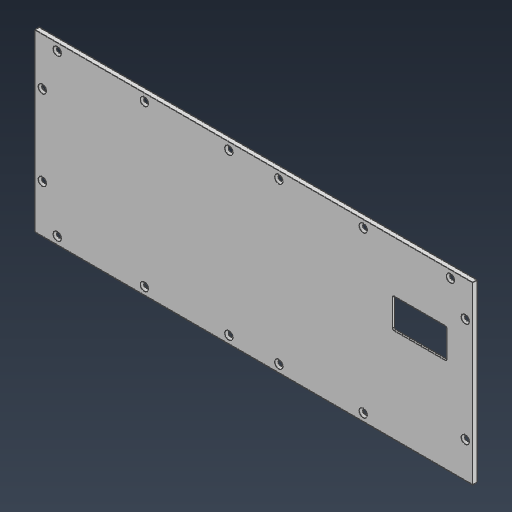
# Autodesk Inventor part: tpu_ceil
Saved by Autodesk Inventor 2023 (Build 270158000, 158)
## iProperties
Created: 2026-01-24
Part Number: tpu_ceil
Material: Generic
Document SubType Name: Modeling
Designer: szymo
Density: 1 g/cm^3
Appearance: Default
Author: szymo
Autodesk Inventor part; units mm, degrees
ref_plane "YZ Plane" through (0, 0, 0) normal (1, 0, 0) x (0, 1, 0)
ref_plane "Work Plane1" through (-125, 0, 3) normal (0, 0, 1) x (1, 0, 0)
sketch "Sketch1" plane through (-125, 0, 3) normal (0, 0, 1) x (1, 0, 0)
  circle A0 centre (241.5, 59.5) radius 1.5 projected
  circle A1 centre (163.8333, 91.5) radius 0.5 projected
  circle A2 centre (28.5, -91.5) radius 2.5 projected
  circle A3 centre (86.1667, -91.5) radius 0.5 projected
  circle A4 centre (125, 91.5) radius 1.5 projected
  circle A5 centre (241.5, 91.5) radius 0.5 projected
  circle A6 centre (241.5, 0) radius 0.5 projected
  circle A7 centre (241.5, -91.5) radius 0.5 projected
  circle A8 centre (28.5, 91.5) radius 1.5 projected
  circle A9 centre (125, -91.5) radius 1.5 projected
  circle A10 centre (86.1667, 91.5) radius 0.5 projected
  circle A11 centre (224.5, 91.5) radius 1.5 projected
  circle A12 centre (241.5, -59.5) radius 1.5 projected
  line L0 (151.825, -90.2) -> (140.325, -90.2) projected
  line L1 (151.825, -97.6) -> (151.825, -90.2) projected
  line L2 (140.325, -97.6) -> (151.825, -97.6) projected
  line L3 (140.325, -90.2) -> (140.325, -97.6) projected
  line L4 (250, -100) -> (0, -100) projected
  line L5 (250, 100) -> (250, -100) projected
  line L6 (0, 100) -> (250, 100) projected
  line L7 (0, 83) -> (0, 100) projected
  line L8 (233, 83) -> (0, 83) projected
  line L9 (233, -83) -> (233, 83) projected
  line L10 (0, -83) -> (233, -83) projected
  line L11 (0, -100) -> (0, -83) projected
  line L12 (197.325, -97.6) -> (208.825, -97.6) projected
  line L13 (197.325, -90.2) -> (197.325, -97.6) projected
  line L14 (208.825, -90.2) -> (197.325, -90.2) projected
  line L15 (208.825, -97.6) -> (208.825, -90.2) projected
  arc A13 (28.5, -96.5) -> (33.5, -91.5) centre (28.5, -91.5) ccw projected
  line L16 (33.5, -91.5) -> (33.5, 91.5) projected
  arc A14 (33.5, 91.5) -> (28.5, 96.5) centre (28.5, 91.5) ccw projected
  line L17 (28.5, 96.5) -> (-28.5, 96.5) projected
  arc A15 (-28.5, 96.5) -> (-33.5, 91.5) centre (-28.5, 91.5) ccw projected
  line L18 (-33.5, 91.5) -> (-33.5, -91.5) projected
  arc A16 (-33.5, -91.5) -> (-28.5, -96.5) centre (-28.5, -91.5) ccw projected
  line L19 (-28.5, -96.5) -> (28.5, -96.5) projected
  circle A17 centre (-28.5, 91.5) radius 1.5 projected
  circle A18 centre (-125, -91.5) radius 1.5 projected
  circle A19 centre (-241.5, 45.75) radius 1.5 projected
  circle A20 centre (-224.5, -91.5) radius 1.5 projected
  circle A21 centre (-241.5, -45.75) radius 1.5 projected
  circle A22 centre (-224.5, 91.5) radius 1.5 projected
  circle A23 centre (-28.5, -91.5) radius 1.5 projected
  circle A24 centre (-125, 91.5) radius 1.5 projected
  circle A25 centre (-163.8333, -91.5) radius 0.5 projected
  circle A26 centre (-241.5, 91.5) radius 0.5 projected
  circle A27 centre (-241.5, -91.5) radius 0.5 projected
  circle A28 centre (-86.1667, -91.5) radius 0.5 projected
  circle A29 centre (-241.5, 0) radius 0.5 projected
  circle A30 centre (-163.8333, 91.5) radius 0.5 projected
  circle A31 centre (-86.1667, 91.5) radius 0.5 projected
  line L20 (-250, 100) -> (-250, -100) projected
  line L21 (-250, -100) -> (0, -100) projected
  line L22 (0, -100) -> (0, -83) projected
  line L23 (0, -83) -> (-233, -83) projected
  line L24 (-233, -83) -> (-233, 83) projected
  line L25 (-233, 83) -> (0, 83) projected
  line L26 (0, 83) -> (0, 100) projected
  line L27 (0, 100) -> (-250, 100) projected
  arc A32 (-246.5, 45.75) -> (-239.7041, 41.0837) centre (-241.5, 45.75) ccw projected
  arc A33 (-239.7041, -41.0837) -> (-239.7041, 41.0837) centre (-233, 0) ccw projected
  arc A34 (-239.7041, -41.0837) -> (-246.5, -45.75) centre (-241.5, -45.75) ccw projected
  line L28 (-246.5, -45.75) -> (-246.5, -91.5) projected
  arc A35 (-246.5, -91.5) -> (-241.5, -96.5) centre (-241.5, -91.5) ccw projected
  line L29 (-241.5, -96.5) -> (-224.5, -96.5) projected
  arc A36 (-224.5, -96.5) -> (-219.5, -91.5) centre (-224.5, -91.5) ccw projected
  arc A37 (-157.8541, -15.573) -> (-219.5, -91.5) centre (-116.6841, -111.9884) ccw projected
  arc A38 (-130, -33.9663) -> (-157.8541, -15.573) centre (-150, -33.9663) ccw projected
  line L30 (-130, -33.9663) -> (-130, -91.5) projected
  arc A39 (-130, -91.5) -> (-120, -91.5) centre (-125, -91.5) ccw projected
  line L31 (-120, -91.5) -> (-120, 91.5) projected
  arc A40 (-120, 91.5) -> (-130, 91.5) centre (-125, 91.5) ccw projected
  line L32 (-130, 91.5) -> (-130, 33.9663) projected
  arc A41 (-157.8541, 15.573) -> (-130, 33.9663) centre (-150, 33.9663) ccw projected
  arc A42 (-219.5, 91.5) -> (-157.8541, 15.573) centre (-116.6841, 111.9884) ccw projected
  arc A43 (-219.5, 91.5) -> (-224.5, 96.5) centre (-224.5, 91.5) ccw projected
  line L33 (-224.5, 96.5) -> (-241.5, 96.5) projected
  arc A44 (-241.5, 96.5) -> (-246.5, 91.5) centre (-241.5, 91.5) ccw projected
  line L34 (-246.5, 91.5) -> (-246.5, 45.75) projected
  line L35 (-28.5, 97.5) -> (28.5, 97.5)
  arc A45 (34.5, 91.5) -> (28.5, 97.5) centre (28.5, 91.5) ccw
  line L36 (34.5, 91.5) -> (34.5, -91.5)
  arc A46 (28.5, -97.5) -> (34.5, -91.5) centre (28.5, -91.5) ccw
  line L37 (28.5, -97.5) -> (-28.5, -97.5)
  arc A47 (-34.5, -91.5) -> (-28.5, -97.5) centre (-28.5, -91.5) ccw
  line L38 (-34.5, -91.5) -> (-34.5, 91.5)
  arc A48 (-28.5, 97.5) -> (-34.5, 91.5) centre (-28.5, 91.5) ccw
  arc A49 (246.5, -59.5) -> (241.5, -54.5) centre (241.5, -59.5) ccw projected
  arc A50 (241.5, 54.5) -> (241.5, -54.5) centre (335.2622, 0) ccw projected
  arc A51 (241.5, 54.5) -> (246.5, 59.5) centre (241.5, 59.5) ccw projected
  line L39 (246.5, 59.5) -> (246.5, 91.5) projected
  arc A52 (246.5, 91.5) -> (241.5, 96.5) centre (241.5, 91.5) ccw projected
  line L40 (241.5, 96.5) -> (224.5, 96.5) projected
  arc A53 (224.5, 96.5) -> (219.5, 91.5) centre (224.5, 91.5) ccw projected
  arc A54 (130, 91.5) -> (219.5, 91.5) centre (174.75, 149.1692) ccw projected
  arc A55 (130, 91.5) -> (120, 91.5) centre (125, 91.5) ccw projected
  line L41 (120, 91.5) -> (120, -91.5) projected
  arc A56 (120, -91.5) -> (130, -91.5) centre (125, -91.5) ccw projected
  arc A57 (184.1388, -71.3462) -> (130, -91.5) centre (241.5, -308.2269) ccw projected
  arc A58 (236.5, -91.5) -> (184.1388, -71.3462) centre (176.2202, -170.0154) ccw projected
  arc A59 (236.5, -91.5) -> (246.5, -91.5) centre (241.5, -91.5) ccw projected
  line L42 (246.5, -91.5) -> (246.5, -59.5) projected
  line L43 (-119, 91.5) -> (-119, -91.5)
  arc A60 (-131, -91.5) -> (-119, -91.5) centre (-125, -91.5) ccw
  line L44 (-131, -91.5) -> (-131, -33.9663)
  arc A61 (-131, -33.9663) -> (-157.4614, -16.4927) centre (-150, -33.9663) ccw
  arc A62 (-157.4614, -16.4927) -> (-218.5009, -91.6034) centre (-116.6841, -111.9884) ccw
  arc A63 (-224.5, -97.5) -> (-218.5009, -91.6034) centre (-224.5, -91.5) ccw
  line L45 (-224.5, -97.5) -> (-241.5, -97.5)
  arc A64 (-247.5, -91.5) -> (-241.5, -97.5) centre (-241.5, -91.5) ccw
  line L46 (-247.5, -91.5) -> (-247.5, -45.75)
  arc A65 (-239.4465, -40.1124) -> (-247.5, -45.75) centre (-241.5, -45.75) ccw
  arc A66 (-239.4465, -40.1124) -> (-239.4465, 40.1124) centre (-233, 0) ccw
  arc A67 (-247.5, 45.75) -> (-239.4465, 40.1124) centre (-241.5, 45.75) ccw
  line L47 (-247.5, 45.75) -> (-247.5, 91.5)
  arc A68 (-241.5, 97.5) -> (-247.5, 91.5) centre (-241.5, 91.5) ccw
  line L48 (-241.5, 97.5) -> (-224.5, 97.5)
  arc A69 (-218.5009, 91.6034) -> (-224.5, 97.5) centre (-224.5, 91.5) ccw
  arc A70 (-218.5009, 91.6034) -> (-157.4614, 16.4927) centre (-116.6841, 111.9884) ccw
  arc A71 (-157.4614, 16.4927) -> (-131, 33.9663) centre (-150, 33.9663) ccw
  line L49 (-131, 33.9663) -> (-131, 91.5)
  arc A72 (-119, 91.5) -> (-131, 91.5) centre (-125, 91.5) ccw
  line L50 (119, -91.5) -> (119, 91.5)
  arc A73 (130.9784, 92.0084) -> (119, 91.5) centre (125, 91.5) ccw
  arc A74 (130.9784, 92.0084) -> (218.5216, 92.0084) centre (174.75, 149.1692) ccw
  arc A75 (224.5, 97.5) -> (218.5216, 92.0084) centre (224.5, 91.5) ccw
  line L51 (224.5, 97.5) -> (241.5, 97.5)
  arc A76 (247.5, 91.5) -> (241.5, 97.5) centre (241.5, 91.5) ccw
  line L52 (247.5, 91.5) -> (247.5, 59.5)
  arc A77 (242.0941, 53.5295) -> (247.5, 59.5) centre (241.5, 59.5) ccw
  arc A78 (242.0941, 53.5295) -> (242.0941, -53.5295) centre (335.2622, 0) ccw
  arc A79 (247.5, -59.5) -> (242.0941, -53.5295) centre (241.5, -59.5) ccw
  line L53 (247.5, -59.5) -> (247.5, -91.5)
  arc A80 (235.5218, -92.0111) -> (247.5, -91.5) centre (241.5, -91.5) ccw
  arc A81 (235.5218, -92.0111) -> (184.2182, -72.3559) centre (176.2202, -170.0154) ccw
  arc A82 (184.2182, -72.3559) -> (130.9671, -92.1278) centre (241.5, -308.2269) ccw
  arc A83 (119, -91.5) -> (130.9671, -92.1278) centre (125, -91.5) ccw
  circle A84 centre (-28.5, 91.5) radius 4 projected
  circle A85 centre (28.5, -91.5) radius 4 projected
  circle A86 centre (-28.5, -91.5) radius 4 projected
  circle A87 centre (28.5, 91.5) radius 4 projected
  circle A88 centre (-224.5, -91.5) radius 4 projected
  circle A89 centre (-241.5, 45.75) radius 4 projected
  circle A90 centre (-125, 91.5) radius 4 projected
  circle A91 centre (-224.5, 91.5) radius 4 projected
  circle A92 centre (-241.5, -45.75) radius 4 projected
  circle A93 centre (-125, -91.5) radius 4 projected
  circle A94 centre (224.5, 91.5) radius 4 projected
  circle A95 centre (125, -91.5) radius 4 projected
  circle A96 centre (241.5, -59.5) radius 4 projected
  circle A97 centre (125, 91.5) radius 4 projected
  circle A98 centre (241.5, 59.5) radius 4 projected
  circle A99 centre (176.2202, -33.9663) radius 26.1144 projected
  circle A100 centre (145.1053, 56.1526) radius 12.5237 projected
  arc A101 (161.2469, 11.514) -> (162.4469, 10.314) centre (162.4469, 11.514) ccw projected
  line L54 (161.2469, 11.514) -> (161.2469, 19.064) projected
  line L55 (161.2469, 19.064) -> (159.9469, 19.064) projected
  line L56 (159.9469, 19.064) -> (159.9469, 29.964) projected
  line L57 (159.9469, 29.964) -> (161.2469, 29.964) projected
  line L58 (161.2469, 29.964) -> (161.2469, 37.514) projected
  arc A102 (162.4469, 38.714) -> (161.2469, 37.514) centre (162.4469, 37.514) ccw projected
  line L59 (162.4469, 38.714) -> (216.4469, 38.714) projected
  arc A103 (217.6469, 37.514) -> (216.4469, 38.714) centre (216.4469, 37.514) ccw projected
  line L60 (217.6469, 37.514) -> (217.6469, 29.964) projected
  line L61 (217.6469, 29.964) -> (218.9469, 29.964) projected
  line L62 (218.9469, 29.964) -> (218.9469, 19.064) projected
  line L63 (218.9469, 19.064) -> (217.6469, 19.064) projected
  line L64 (217.6469, 19.064) -> (217.6469, 11.514) projected
  arc A104 (216.4469, 10.314) -> (217.6469, 11.514) centre (216.4469, 11.514) ccw projected
  line L65 (216.4469, 10.314) -> (162.4469, 10.314) projected
  arc A105 (159.4469, 9.014) -> (159.9469, 8.514) centre (159.9469, 9.014) ccw projected
  line L66 (159.9469, 8.514) -> (218.9469, 8.514) projected
  arc A106 (218.9469, 8.514) -> (219.4469, 9.014) centre (218.9469, 9.014) ccw projected
  line L67 (219.4469, 9.014) -> (219.4469, 40.014) projected
  arc A107 (219.4469, 40.014) -> (218.9469, 40.514) centre (218.9469, 40.014) ccw projected
  line L68 (218.9469, 40.514) -> (159.9469, 40.514) projected
  arc A108 (159.9469, 40.514) -> (159.4469, 40.014) centre (159.9469, 40.014) ccw projected
  line L69 (159.4469, 40.014) -> (159.4469, 9.014) projected
  line L70 (160.9469, 10.014) -> (217.9469, 10.014) projected
  arc A109 (160.4469, 10.514) -> (160.9469, 10.014) centre (160.9469, 10.514) ccw projected
  line L71 (160.4469, 38.514) -> (160.4469, 10.514) projected
  arc A110 (160.9469, 39.014) -> (160.4469, 38.514) centre (160.9469, 38.514) ccw projected
  line L72 (217.9469, 39.014) -> (160.9469, 39.014) projected
  arc A111 (218.4469, 38.514) -> (217.9469, 39.014) centre (217.9469, 38.514) ccw projected
  line L73 (218.4469, 10.514) -> (218.4469, 38.514) projected
  arc A112 (217.9469, 10.014) -> (218.4469, 10.514) centre (217.9469, 10.514) ccw projected
  line L74 (218.9469, 7.514) -> (159.9469, 7.514)
  arc A113 (158.4469, 9.014) -> (159.9469, 7.514) centre (159.9469, 9.014) ccw
  line L75 (158.4469, 9.014) -> (158.4469, 40.014)
  arc A114 (159.9469, 41.514) -> (158.4469, 40.014) centre (159.9469, 40.014) ccw
  line L76 (159.9469, 41.514) -> (218.9469, 41.514)
  arc A115 (220.4469, 40.014) -> (218.9469, 41.514) centre (218.9469, 40.014) ccw
  line L77 (220.4469, 40.014) -> (220.4469, 9.014)
  arc A116 (218.9469, 7.514) -> (220.4469, 9.014) centre (218.9469, 9.014) ccw
  point P0 (125, 0)
  dimension "d0" = 1
  dimension "d1" = 1
  dimension "d2" = 1
  dimension "d15" = 1
  constraints: 64 point on circle, 38 end point, 32 centre point, 47 other
  measures "d0" distance between parallel lines of L17 L35
  measures "d1" distance between parallel lines of L31 L43
  measures "d2" distance between parallel lines of L41 L50
  measures "d15" distance between parallel lines of L66 L74
ref_plane "Work Plane2" through (-375, -100, 0) normal (0, 0, 1) x (1, 0, 0)
extrude "Extrusion1" add sketch "Sketch1" against normal up to surface (3 mm away) contours A1 | A3 | A6 | A10 | L1 L2 L3 L0 | L4 L11 L37 A46 L36 L10 L50 A83 A82 A81 A80 L53 A79 A78 L9 A77 L52 A76 L51 A75 A74 L8 A73 A45 L35 L7 L6 L5 | L21 L20 L27 L7 L35 A48 L38 L25 L43 A72 L49 A70 A69 L48 A68 L47 A67 A66 L24 A65 L46 A64 L45 A63 A62 L23 L44 A60 A47 L37 L11 | L36 L8 L50 L10 | L23 L43 L25 L38 | A82 A81 L10 | L23 A62 A61 L44 | L8 A74 | L49 A71 A70 L25 | A78 L9 | L24 A66 | L13 L14 L15 L12 | A25 | A28 | A29 | A30 | A31
sketch "Sketch2" plane through (-125, 0, 3) normal (0, 0, 1) x (1, 0, 0)
  line L0 (-250, 100) -> (-250, -100) projected
  line L1 (-250, -100) -> (250, -100) projected
  line L2 (250, -100) -> (250, 100) projected
  line L3 (250, 100) -> (-250, 100) projected
  line L4 (34.5, 91.5) -> (34.5, -91.5) projected
  arc A0 (28.5, -97.5) -> (34.5, -91.5) centre (28.5, -91.5) ccw projected
  line L5 (28.5, -97.5) -> (-28.5, -97.5) projected
  arc A1 (-34.5, -91.5) -> (-28.5, -97.5) centre (-28.5, -91.5) ccw projected
  line L6 (-34.5, -91.5) -> (-34.5, 91.5) projected
  arc A2 (-28.5, 97.5) -> (-34.5, 91.5) centre (-28.5, 91.5) ccw projected
  line L7 (-28.5, 97.5) -> (28.5, 97.5) projected
  arc A3 (34.5, 91.5) -> (28.5, 97.5) centre (28.5, 91.5) ccw projected
  line L8 (119, -91.5) -> (119, 91.5) projected
  arc A4 (130.9784, 92.0084) -> (119, 91.5) centre (125, 91.5) ccw projected
  arc A5 (130.9784, 92.0084) -> (218.5216, 92.0084) centre (174.75, 149.1692) ccw projected
  arc A6 (224.5, 97.5) -> (218.5216, 92.0084) centre (224.5, 91.5) ccw projected
  line L9 (224.5, 97.5) -> (241.5, 97.5) projected
  arc A7 (247.5, 91.5) -> (241.5, 97.5) centre (241.5, 91.5) ccw projected
  line L10 (247.5, 91.5) -> (247.5, 59.5) projected
  arc A8 (242.0941, 53.5295) -> (247.5, 59.5) centre (241.5, 59.5) ccw projected
  arc A9 (242.0941, 53.5295) -> (242.0941, -53.5295) centre (335.2622, 0) ccw projected
  arc A10 (247.5, -59.5) -> (242.0941, -53.5295) centre (241.5, -59.5) ccw projected
  line L11 (247.5, -59.5) -> (247.5, -91.5) projected
  arc A11 (235.5218, -92.0111) -> (247.5, -91.5) centre (241.5, -91.5) ccw projected
  arc A12 (235.5218, -92.0111) -> (184.2182, -72.3559) centre (176.2202, -170.0154) ccw projected
  arc A13 (184.2182, -72.3559) -> (130.9671, -92.1278) centre (241.5, -308.2269) ccw projected
  arc A14 (119, -91.5) -> (130.9671, -92.1278) centre (125, -91.5) ccw projected
  line L12 (-119, 91.5) -> (-119, -91.5) projected
  arc A15 (-131, -91.5) -> (-119, -91.5) centre (-125, -91.5) ccw projected
  line L13 (-131, -91.5) -> (-131, -33.9663) projected
  arc A16 (-131, -33.9663) -> (-157.4614, -16.4927) centre (-150, -33.9663) ccw projected
  arc A17 (-157.4614, -16.4927) -> (-218.5009, -91.6034) centre (-116.6841, -111.9884) ccw projected
  arc A18 (-224.5, -97.5) -> (-218.5009, -91.6034) centre (-224.5, -91.5) ccw projected
  line L14 (-224.5, -97.5) -> (-241.5, -97.5) projected
  arc A19 (-247.5, -91.5) -> (-241.5, -97.5) centre (-241.5, -91.5) ccw projected
  line L15 (-247.5, -91.5) -> (-247.5, -45.75) projected
  arc A20 (-239.4465, -40.1124) -> (-247.5, -45.75) centre (-241.5, -45.75) ccw projected
  arc A21 (-239.4465, -40.1124) -> (-239.4465, 40.1124) centre (-233, 0) ccw projected
  arc A22 (-247.5, 45.75) -> (-239.4465, 40.1124) centre (-241.5, 45.75) ccw projected
  line L16 (-247.5, 45.75) -> (-247.5, 91.5) projected
  arc A23 (-241.5, 97.5) -> (-247.5, 91.5) centre (-241.5, 91.5) ccw projected
  line L17 (-241.5, 97.5) -> (-224.5, 97.5) projected
  arc A24 (-218.5009, 91.6034) -> (-224.5, 97.5) centre (-224.5, 91.5) ccw projected
  arc A25 (-218.5009, 91.6034) -> (-157.4614, 16.4927) centre (-116.6841, 111.9884) ccw projected
  arc A26 (-157.4614, 16.4927) -> (-131, 33.9663) centre (-150, 33.9663) ccw projected
  line L18 (-131, 33.9663) -> (-131, 91.5) projected
  arc A27 (-119, 91.5) -> (-131, 91.5) centre (-125, 91.5) ccw projected
  line L19 (250, 100) -> (250, -100) projected
  line L20 (250, 100) -> (-250, 100)
  line L21 (-250, 100) -> (-250, -100)
  line L22 (-250, -100) -> (250, -100)
  line L23 (250, -100) -> (250, 100)
  arc A28 (159.4469, 9.014) -> (159.9469, 8.514) centre (159.9469, 9.014) ccw projected
  line L24 (159.9469, 8.514) -> (218.9469, 8.514) projected
  arc A29 (218.9469, 8.514) -> (219.4469, 9.014) centre (218.9469, 9.014) ccw projected
  line L25 (219.4469, 9.014) -> (219.4469, 40.014) projected
  arc A30 (219.4469, 40.014) -> (218.9469, 40.514) centre (218.9469, 40.014) ccw projected
  line L26 (218.9469, 40.514) -> (159.9469, 40.514) projected
  arc A31 (159.9469, 40.514) -> (159.4469, 40.014) centre (159.9469, 40.014) ccw projected
  line L27 (159.4469, 40.014) -> (159.4469, 9.014) projected
  line L28 (160.9469, 10.014) -> (217.9469, 10.014) projected
  arc A32 (160.4469, 10.514) -> (160.9469, 10.014) centre (160.9469, 10.514) ccw projected
  line L29 (160.4469, 38.514) -> (160.4469, 10.514) projected
  arc A33 (160.9469, 39.014) -> (160.4469, 38.514) centre (160.9469, 38.514) ccw projected
  line L30 (217.9469, 39.014) -> (160.9469, 39.014) projected
  arc A34 (218.4469, 38.514) -> (217.9469, 39.014) centre (217.9469, 38.514) ccw projected
  line L31 (218.4469, 10.514) -> (218.4469, 38.514) projected
  arc A35 (217.9469, 10.014) -> (218.4469, 10.514) centre (217.9469, 10.514) ccw projected
  line L32 (218.9469, 7.514) -> (159.9469, 7.514)
  arc A36 (158.4469, 9.014) -> (159.9469, 7.514) centre (159.9469, 9.014) ccw
  line L33 (158.4469, 9.014) -> (158.4469, 40.014)
  arc A37 (159.9469, 41.514) -> (158.4469, 40.014) centre (159.9469, 40.014) ccw
  line L34 (159.9469, 41.514) -> (218.9469, 41.514)
  arc A38 (220.4469, 40.014) -> (218.9469, 41.514) centre (218.9469, 40.014) ccw
  line L35 (220.4469, 40.014) -> (220.4469, 9.014)
  arc A39 (218.9469, 7.514) -> (220.4469, 9.014) centre (218.9469, 9.014) ccw
  point P0 (125, 0)
  dimension "d16" = 1
  constraints: 16 end point, 8 point on circle, 4 centre point, 2 parallel, 1 horizontal, 1 perpendicular, 7 other
  measures "d16" distance between parallel lines of L24 L32
extrude "Extrusion2" add sketch "Sketch2" along normal blind 2 contours L3 L2 L1 L0 | L4 A0 L5 A1 L6 A2 L7 A3 | L8 A4 A5 A6 L9 A7 L10 A8 A9 A10 L11 A11 A12 A13 A14 | L12 A15 L13 A16 A17 A18 L14 A19 L15 A20 A21 A22 L16 A23 L17 A24 A25 A26 L18 A27
sketch "Sketch3" plane through (-125, 0, 5) normal (0, 0, 1) x (1, 0, 0)
  circle A0 centre (241.5, -59.5) radius 2.5 projected
  circle A1 centre (241.5, 59.5) radius 2.5 projected
  circle A2 centre (224.5, 91.5) radius 2.5 projected
  circle A3 centre (125, 91.5) radius 2.5 projected
  circle A4 centre (28.5, 91.5) radius 2.5 projected
  circle A5 centre (-28.5, 91.5) radius 2.5 projected
  circle A6 centre (-125, 91.5) radius 2.5 projected
  circle A7 centre (-224.5, 91.5) radius 2.5 projected
  circle A8 centre (-241.5, 45.75) radius 2.5 projected
  circle A9 centre (-241.5, -45.75) radius 2.5 projected
  circle A10 centre (-224.5, -91.5) radius 2.5 projected
  circle A11 centre (-125, -91.5) radius 2.5 projected
  circle A12 centre (-28.5, -91.5) radius 2.5 projected
  circle A13 centre (28.5, -91.5) radius 2.5 projected
  circle A14 centre (125, -91.5) radius 2.5 projected
  point P0 (125, 0)
hole "Hole1" at (-366.5, 45.75, 5) at (-349.5, 91.5, 5) at (-366.5, -45.75, 5) at (-349.5, -91.5, 5) at (-250, 91.5, 5) at (-250, -91.5, 5) at (-153.5, -91.5, 5) at (-153.5, 91.5, 5) at (-96.5, 91.5, 5) at (-96.5, -91.5, 5) at (0, 91.5, 5) at (0, -91.5, 5) at (116.5, -59.5, 5) at (116.5, 59.5, 5) at (99.5, 91.5, 5) direction (0, 0, -1) diameter 4.5 end through all countersink diameter 9.5 countersink angle 90 clearance for "Countersunk Flat Head Screw ISO 2009/7046" size "M4" standard "ISO"
body "Solid1"
